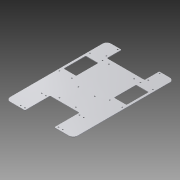
# Autodesk Inventor part: Board 1
Saved by Autodesk Inventor 2015 (Build 190159000, 159)
## iProperties
Created: 2015-05-24
Part Number: Board 1
Material: アルミニウム 6061
Document SubType Name: Modeling
Designer: kenta
Density: 2.7 g/cm^3
Appearance: アルミニウム - フラット - Version 1.1
Mass: 111.881 g
Surface Area: 575.08 cm^2
Volume: 41.4375 cm^3
Author: kenta
Autodesk Inventor part; units mm, degrees
ref_plane "YZ Plane" through (0, 0, 0) normal (1, 0, 0) x (0, 1, 0)
ref_plane "XZ Plane" through (0, 0, 0) normal (0, 1, 0) x (-1, 0, 0)
ref_plane "XY Plane" through (0, 0, 0) normal (0, 0, 1) x (1, 0, 0)
sketch "スケッチ1" plane through (0, 0, 0) normal (0, 0, 1) x (1, 0, 0)
  line L0 (80, 100) -> (-80, 100)
  line L1 (-80, 100) -> (-80, -100)
  line L2 (-80, -100) -> (80, -100)
  line L3 (80, -100) -> (80, 100)
  line L4 (80, 100) -> (-80, -100) construction
  line L5 (-80, 100) -> (80, -100) construction
  point P0 (0, 0)
  dimension "d0" = 160
  dimension "d1" = 200
  constraints: 12 end point, 2 midpoint, 2 parallel, 1 horizontal, 1 perpendicular
  measures "d0" distance of L2.end L1.end
  measures "d1" distance of L1.end L0.end
extrude "押し出し1" add sketch "スケッチ1" along normal blind 1.5
sketch "スケッチ2" plane through (0, 0, 1.5) normal (0, 0, 1) x (1, 0, 0)
  line L0 (80, -100) -> (80, 100) projected
  line L1 (80, 100) -> (-80, 100) projected
  line L2 (-80, 100) -> (-80, -100) projected
  point P0 (0, 0)
  point P1 (-45, 95)
  point P2 (-75, 95)
  point P3 (-75, 22)
  point P4 (-45, 22)
  point P5 (45, 95)
  point P6 (75, 95)
  point P7 (45, 22)
  point P8 (75, 22)
  dimension "d12" = 5
  dimension "d13" = 5
  dimension "d14" = 5
  dimension "d15" = 30
  dimension "d16" = 5
  dimension "d20" = 73
  dimension "d23" = 73
  dimension "d24" = 30
  dimension "d26" = 5
  dimension "d35" = 5
  dimension "d128" = 35
  dimension "d129" = 35
  constraints: 3 horizontal alignment, 1 vertical alignment
  measures "d12" distance from line of point (-75, 95) L1
  measures "d13" distance from line of L2 point (-75, 95)
  measures "d14" distance from line of L1 point (-45, 95)
  measures "d15" distance of point (-75, 95) point (-45, 95)
  measures "d16" distance from line of L2 point (-75, 22)
  measures "d20" distance of point (-45, 95) point (-45, 22)
  measures "d23" distance of point (75, 22) point (75, 95)
  measures "d24" distance of point (45, 95) point (75, 95)
  measures "d26" distance from line of point (75, 95) L0
  measures "d35" distance from line of L1 point (45, 95)
  measures "d128" distance from line of point (-45, 22) L2
  measures "d129" distance from line of point (45, 22) L0
hole "穴1" at (-45, 95, 1.5) at (-75, 95, 1.5) at (-75, 22, 1.5) at (-45, 22, 1.5) at (45, 95, 1.5) at (75, 95, 1.5) at (45, 22, 1.5) at (75, 22, 1.5) direction (0, 0, -1) diameter 3.1 end through all
sketch "スケッチ4" plane through (0, 0, 1.5) normal (0, 0, 1) x (1, 0, 0)
  line L0 (-75, 85) -> (-45, 85)
  line L1 (-45, 85) -> (-45, 32)
  line L2 (-45, 32) -> (-75, 32)
  line L3 (-75, 32) -> (-75, 85)
  line L4 (45, 85) -> (75, 85)
  line L5 (75, 85) -> (75, 32)
  line L6 (75, 32) -> (45, 32)
  line L7 (45, 32) -> (45, 85)
  line L8 (-80, 100) -> (-80, -100) projected
  line L9 (80, -100) -> (80, 100) projected
  line L10 (80, 100) -> (-80, 100) projected
  point P0 (0, 0)
  dimension "d46" = 30
  dimension "d47" = 53
  dimension "d48" = 30
  dimension "d49" = 53
  dimension "d50" = 5
  dimension "d51" = 5
  dimension "d52" = 15
  dimension "d53" = 15
  constraints: 16 end point, 4 parallel, 2 horizontal, 2 perpendicular
  measures "d46" distance of L1.end L2.end
  measures "d47" distance of L0.end L1.end
  measures "d48" distance of L5.end L6.end
  measures "d49" distance of L4.end L5.end
  measures "d50" distance between parallel lines of L3 L8
  measures "d51" distance between parallel lines of L5 L9
  measures "d52" distance between parallel lines of L4 L10
  measures "d53" distance between parallel lines of L0 L10
extrude "押し出し2" cut sketch "スケッチ4" against normal blind 1.5
fillet "フィレット1" radius 2 8 edges at (-75, 85, 0.75) (-45, 85, 0.75) (75, 85, 0.75) (45, 85, 0.75) (-75, 32, 0.75) (45, 32, 0.75) (-45, 32, 0.75) (75, 32, 0.75)
sketch "スケッチ5" plane through (0, 0, 1.5) normal (0, 0, 1) x (1, 0, 0)
  line L0 (-35, -40) -> (35, -40)
  line L1 (35, -40) -> (35, -100)
  line L2 (35, -100) -> (-35, -100)
  line L3 (-35, -100) -> (-35, -40)
  line L4 (-80, -100) -> (80, -100) projected
  point P0 (0, 0)
  dimension "d57" = 70
  dimension "d58" = 60
  dimension "d59" = 35
  dimension "d60" = 0
  constraints: 8 end point, 2 parallel, 1 horizontal, 1 perpendicular
  measures "d57" distance of L1.end L2.end
  measures "d58" distance of L0.end L1.end
  measures "d59" distance from line of point (0, 0) L3
  measures "d60" distance between parallel lines of L2 L4
extrude "押し出し3" cut sketch "スケッチ5" against normal blind 1.5
sketch "スケッチ6" plane through (0, 0, 1.5) normal (0, 0, 1) x (1, 0, 0)
  line L0 (35, -40) -> (35, -100) projected
  line L1 (-35, -100) -> (-35, -40) projected
  line L2 (35, -100) -> (80, -100) projected
  line L3 (-35, -40) -> (35, -40) projected
  point P0 (0, 0)
  point P1 (40, -95)
  point P2 (40, -45)
  point P3 (-40, -45)
  point P4 (-40, -95)
  point P5 (50, -45)
  point P6 (50, -95)
  point P7 (-50, -45)
  point P8 (-50, -95)
  dimension "d63" = 5
  dimension "d64" = 5
  dimension "d65" = 5
  dimension "d66" = 5
  dimension "d84" = 10
  dimension "d85" = 10
  dimension "d86" = 50
  dimension "d87" = 50
  dimension "d88" = 10
  dimension "d89" = 10
  dimension "d90" = 45
  constraints: 2 horizontal alignment, 2 vertical alignment
  measures "d63" distance from line of point (40, -95) L0
  measures "d64" distance from line of point (-40, -95) L1
  measures "d65" distance from line of point (40, -95) L2
  measures "d66" distance from line of point (40, -45) L3
  measures "d84" distance of point (50, -95) point (40, -95)
  measures "d85" distance of point (40, -45) point (50, -45)
  measures "d86" distance of point (50, -95) point (50, -45)
  measures "d87" distance of point (-50, -95) point (-50, -45)
  measures "d88" distance of point (-50, -45) point (-40, -45)
  measures "d89" distance of point (-40, -95) point (-50, -95)
  measures "d90" vertical distance of point (0, 0) point (-50, -45)
hole "穴3" at (40, -95, 1.5) at (40, -45, 1.5) at (-40, -45, 1.5) at (-40, -95, 1.5) at (50, -45, 1.5) at (50, -95, 1.5) at (-50, -95, 1.5) at (-50, -45, 1.5) direction (0, 0, -1) diameter 3.1 end through all
sketch "スケッチ7" plane through (0, 0, 1.5) normal (0, 0, 1) x (1, 0, 0)
  line L0 (80, 100) -> (-80, 100) projected
  point P0 (0, 0)
  point P1 (-30, 95)
  point P2 (30, 95)
  dimension "d74" = 5
  dimension "d75" = 60
  dimension "d76" = 30
  constraints: 1 horizontal alignment
  measures "d74" distance from line of point (-30, 95) L0
  measures "d75" distance of point (30, 95) point (-30, 95)
  measures "d76" horizontal distance of point (-30, 95) point (0, 0)
hole "穴4" at (-30, 95, 1.5) at (30, 95, 1.5) direction (0, 0, -1) diameter 3.1 end through all
sketch "スケッチ10" plane through (-80, 100, 0) normal (0, 1, 0) x (1, 0, 0)
  line L0 (160, 0) -> (0, 0)
  line L1 (0, 0) -> (0, -1.5)
  line L2 (0, -1.5) -> (160, -1.5)
  line L3 (160, -1.5) -> (160, 0)
  point P0 (80, 0)
  dimension "d105" = 160
  dimension "d106" = 1.5
  constraints: 8 end point, 2 parallel, 1 horizontal, 1 perpendicular
  measures "d105" distance of L2.end L1.end
  measures "d106" distance of L1.end L0.end
extrude "押し出し4" add sketch "スケッチ10" along normal blind 40
sketch "スケッチ11" plane through (0, 0, 1.5) normal (0, 0, 1) x (1, 0, 0)
  line L0 (45, 140) -> (-45, 140)
  line L1 (-45, 140) -> (-45, 105)
  line L2 (-45, 105) -> (45, 105)
  line L3 (45, 105) -> (45, 140)
  line L4 (-80, 140) -> (80, 140) projected
  line L5 (80, -100) -> (80, 140) projected
  point P0 (0, 0)
  dimension "d109" = 90
  dimension "d110" = 35
  dimension "d111" = 0
  dimension "d112" = 35
  constraints: 8 end point, 2 parallel, 1 horizontal, 1 perpendicular
  measures "d109" distance of L2.end L1.end
  measures "d110" distance of L1.end L0.end
  measures "d111" distance between parallel lines of L4 L0
  measures "d112" distance between parallel lines of L5 L3
extrude "押し出し5" cut sketch "スケッチ11" against normal blind 20
sketch "スケッチ12" plane through (0, 0, 1.5) normal (0, 0, 1) x (1, 0, 0)
  line L0 (45, 140) -> (45, 105) projected
  line L1 (-45, 105) -> (-45, 140) projected
  line L2 (-80, 140) -> (-45, 140) projected
  line L3 (45, 140) -> (80, 140) projected
  point P0 (0, 0)
  point P1 (-50, 136)
  point P2 (-50, 109)
  point P3 (50, 136)
  point P4 (50, 109)
  dimension "d115" = 5
  dimension "d116" = 5
  dimension "d117" = 4
  dimension "d118" = 27
  dimension "d119" = 4
  dimension "d120" = 27
  constraints: 2 vertical alignment
  measures "d115" distance from line of point (50, 136) L0
  measures "d116" distance from line of point (-50, 136) L1
  measures "d117" distance from line of point (-50, 136) L2
  measures "d118" distance of point (-50, 109) point (-50, 136)
  measures "d119" distance from line of point (50, 136) L3
  measures "d120" distance of point (50, 136) point (50, 109)
hole "穴6" at (-50, 136, 1.5) at (-50, 109, 1.5) at (50, 136, 1.5) at (50, 109, 1.5) direction (0, 0, -1) diameter 3.1 depth 8 tip angle 118
fillet "フィレット4" radius 10 4 edges at (80, 140, 0.75) (-80, 140, 0.75) (-80, -100, 0.75) (80, -100, 0.75)
fillet "フィレット5" radius 2 8 edges at (-45, 105, 0.75) (-45, 140, 0.75) (45, 105, 0.75) (45, 140, 0.75) (-35, -40, 0.75) (35, -40, 0.75) (-35, -100, 0.75) (35, -100, 0.75)
sketch "スケッチ13" plane through (0, 0, 1.5) normal (0, 0, 1) x (1, 0, 0)
  line L0 (-80, -90) -> (-80, 130) projected
  circle A0 centre (-45, 22) radius 1.55 projected
  point P0 (0, 0)
  point P1 (-19.5, -33)
  point P2 (19.5, -33)
  point P3 (-19.5, 12)
  point P4 (19.5, 12)
  dimension "d134" = 39
  dimension "d135" = 45
  dimension "d136" = 60.5
  dimension "d137" = 10
  constraints: 2 horizontal alignment, 2 vertical alignment
  measures "d134" distance of point (19.5, 12) point (-19.5, 12)
  measures "d135" distance of point (19.5, 12) point (19.5, -33)
  measures "d136" distance from line of point (-19.5, 12) L0
  measures "d137" vertical distance of A0.centre point (-19.5, 12)
hole "穴7" at (-19.5, -33, 1.5) at (19.5, -33, 1.5) at (-19.5, 12, 1.5) at (19.5, 12, 1.5) direction (0, 0, -1) diameter 3 end through all
